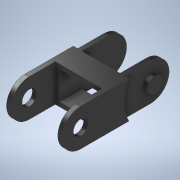
# Autodesk Inventor part: cadena_link_terminal
Saved by Autodesk Inventor 2021 (Build 250183000, 183)
## iProperties
Created: 2021-06-22
Part Number: cadena_link_terminal
Material: Plástico PC/ABS
Document SubType Name: Modeling
Designer: Leonardo Fabio Mercado Benítez
Density: 0.357273 g/cm^3
Appearance: Suave - Blanco
Author: Leonardo Fabio Mercado Benítez
Autodesk Inventor part; units mm, degrees
ref_plane "YZ Plane" through (0, 0, 0) normal (1, 0, 0) x (0, 1, 0)
ref_plane "XZ Plane" through (0, 0, 0) normal (0, 1, 0) x (-1, 0, 0)
ref_plane "XY Plane" through (0, 0, 0) normal (0, 0, 1) x (1, 0, 0)
sketch "Boceto1" plane through (0, 0, 0) normal (0, 1, 0) x (-1, 0, 0)
  line L0 (-9.525, 19.05) -> (9.525, 19.05)
  line L1 (9.525, 19.05) -> (9.525, -19.05)
  line L2 (9.525, -19.05) -> (-9.525, -19.05)
  line L3 (-9.525, -19.05) -> (-9.525, 19.05)
  line L4 (-9.525, 19.05) -> (9.525, -19.05) construction
  line L5 (9.525, 19.05) -> (-9.525, -19.05) construction
  point P0 (0, 0)
  dimension "d0" = 19.05
  dimension "d1" = 38.1
  constraints: 12 end point, 2 midpoint, 2 parallel, 1 horizontal, 1 perpendicular
  measures "d0" distance of L1.end L2.end
  measures "d1" distance of L0.end L1.end
extrude "Extrusión1" add sketch "Boceto1" along normal blind 12.7
sketch "Boceto3" plane through (9.525, 0, 19.05) normal (1, 0, 0) x (0, 0, -1)
  line L0 (38.1, 0) -> (38.1, 12.7)
  line L1 (38.1, 6.35) -> (38.1, 6.35)
  line L2 (0, 6.35) -> (0, 6.35)
  arc A0 (6.35, 12.7) -> (0, 6.35) centre (6.35, 6.35) ccw
  arc A1 (0, 6.35) -> (6.35, 0) centre (6.35, 6.35) ccw
  arc A2 (38.1, 6.35) -> (31.75, 12.7) centre (31.75, 6.35) ccw
  arc A3 (31.75, 0) -> (38.1, 6.35) centre (31.75, 6.35) ccw
  line L3 (0, 0) -> (0, 12.7)
  line L4 (38.1, 0) -> (31.75, 0)
  line L5 (6.35, 0) -> (0, 0)
  line L6 (0, 12.7) -> (6.35, 12.7)
  line L7 (31.75, 12.7) -> (38.1, 12.7)
  point P0 (19.05, 0)
  point P1 (0, 6.35)
  dimension "d7" = 6.35
  constraints: 16 end point, 8 point on circle, 4 centre point, 4 tangent, 3 equal radius, 2 point on line, 1 parallel
  measures "d7" radius of A0
extrude "Extrusión3" cut sketch "Boceto3" against normal up to surface (19.05 mm away)
sketch "Boceto5" plane through (0, 12.7, 0) normal (0, 1, 0) x (1, 0, 0)
  line L0 (-9.525, 19.05) -> (-9.525, -19.05) projected
  line L1 (9.525, -12.7) -> (9.525, 12.7) projected
  line L2 (9.525, -19.05) -> (9.525, -12.7) projected
  line L3 (-8.025, -3.843) -> (-8.025, -19.05)
  line L4 (8.025, -3.843) -> (8.025, -12.7)
  line L5 (8.025, -12.7) -> (8.025, -19.05)
  line L6 (-8.025, -3.843) -> (8.025, -3.843)
  line L7 (-8.025, -19.05) -> (8.025, -19.05)
  line L8 (-9.525, -19.05) -> (9.525, -19.05) projected
  point P0 (0, 0)
  dimension "d11" = 1.5
  dimension "d12" = 1.5
  constraints: 10 end point, 1 collinear, 1 parallel, 1 perpendicular
  measures "d11" distance between parallel lines of L0 L3
  measures "d12" distance between parallel lines of L1 L4
extrude "Extrusión4" cut sketch "Boceto5" against normal up to surface (12.7 mm away)
sketch "Boceto6" plane through (9.525, 0, 12.7) normal (1, 0, 0) x (0, 0, -1)
  arc A0 (0, 12.7) -> (0, 0) centre (0, 6.35) ccw projected
  circle A1 centre (0, 6.35) radius 2.54
  point P0 (12.7, 0)
  dimension "d15" = 5.08
  constraints: 1 centre point, 1 coincident
  measures "d15" diameter of A1
extrude "Extrusión5" cut sketch "Boceto6" against normal up to surface (19.05 mm away)
sketch "Boceto7" plane through (9.525, 0, 12.7) normal (1, 0, 0) x (0, 0, -1)
  line L0 (0, 12.7) -> (25.4, 12.7) projected
  arc A0 (16.5105, 12.7) -> (16.5105, 0) centre (27.5091, 6.35) ccw
  line L1 (16.5105, 12.7) -> (35.1863, 12.7)
  line L2 (35.1863, 12.7) -> (35.1863, 0)
  line L3 (35.1863, 0) -> (16.5105, 0)
  circle A1 centre (25.4, 6.35) radius 2.54
  point P0 (12.7, 0)
  dimension "d18" = 12.7
  dimension "d19" = 5.08
  constraints: 6 end point, 2 centre point, 2 perpendicular, 2 point on circle, 1 coincident, 1 horizontal, 1 point on line
  measures "d18" radius of A0
  measures "d19" diameter of A1
extrude "Extrusión6" cut sketch "Boceto7" against normal blind 1.5
sketch "Boceto8" plane through (-9.525, 0, -12.7) normal (-1, 0, 0) x (0, 0, 1)
  arc A0 (8.8895, 0) -> (8.8895, 12.7) centre (-2.1091, 6.35) ccw projected
  line L0 (-6.35, 12.7) -> (31.75, 12.7) projected
  line L1 (0, 0) -> (25.4, 0) projected
  circle A1 centre (0, 6.35) radius 2.54 projected
  line L2 (0, 0) -> (-7.3331, 0)
  line L3 (-7.3331, 0) -> (-7.3331, 12.7)
  line L4 (-7.3331, 12.7) -> (-6.35, 12.7)
  point P0 (12.7, 0)
  constraints: 6 end point, 2 perpendicular, 1 horizontal
extrude "Extrusión7" cut sketch "Boceto8" against normal blind 1.5
sketch "Boceto9" plane through (-8.025, 12.7, 3.843) normal (0, 0, 1) x (1, 0, 0)
  line L0 (16.05, -12.7) -> (0, -12.7) projected
  line L1 (16.05, 0) -> (16.05, -12.7) projected
  line L2 (0, 0) -> (16.05, 0) projected
  line L3 (0, 0) -> (0, -12.7) projected
  line L4 (14.55, -1.5) -> (14.55, -11.2)
  line L5 (14.55, -11.2) -> (1.5, -11.2)
  line L6 (1.5, -11.2) -> (1.5, -1.5)
  line L7 (1.5, -1.5) -> (14.55, -1.5)
  point P0 (8.025, -12.7)
  dimension "d24" = 1.5
  constraints: 8 end point, 3 other
  measures "d24" distance between parallel lines of L2 L7
extrude "Extrusión8" cut sketch "Boceto9" against normal blind 25 contours L4 L5 L6 L7
sketch "Boceto10" plane through (0, 12.7, 0) normal (0, 1, 0) x (1, 0, 0)
  line L0 (6.525, 16.7988) -> (-6.525, 16.7988) projected
  line L1 (6.525, 16.7988) -> (6.525, 3.7495)
  line L2 (6.525, -3.843) -> (6.525, 16.7988) projected
  line L3 (-6.525, -3.843) -> (-6.525, 16.7988) projected
  line L4 (-6.525, 3.7495) -> (-6.525, 16.7988)
  line L5 (-6.525, 16.7988) -> (6.525, 16.7988)
  line L6 (-6.525, 3.7495) -> (6.525, 3.7495)
  point P0 (0, 0)
  constraints: 8 end point, 2 point on line, 1 collinear, 1 horizontal, 1 perpendicular
extrude "Extrusión9" cut sketch "Boceto10" against normal up to surface (12.7 mm away)
